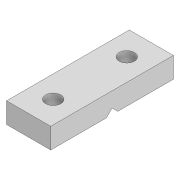
# Autodesk Inventor part: suction_electrode_holder
Saved by Autodesk Inventor 2020 (Build 240168000, 168)
## iProperties
Created: 2020-06-24
Part Number: suction_electrode_holder
Material: Generic
Document SubType Name: Modeling
Designer: Daniel
Density: 1 g/cm^3
Appearance: Default
Author: Daniel
Autodesk Inventor part; units mm, degrees
ref_plane "YZ Plane" through (0, 0, 0) normal (1, 0, 0) x (0, 1, 0)
ref_plane "XZ Plane" through (0, 0, 0) normal (0, 1, 0) x (-1, 0, 0)
ref_plane "XY Plane" through (0, 0, 0) normal (0, 0, 1) x (1, 0, 0)
sketch "Sketch1" plane through (0, 0, 0) normal (0, 1, 0) x (-1, 0, 0)
  line L0 (0, 0) -> (9, 0)
  line L1 (9, 0) -> (9, -25)
  line L2 (9, -25) -> (0, -25)
  line L3 (0, -25) -> (0, 0)
  circle A0 centre (4.5, -5) radius 1.55
  circle A1 centre (4.5, -20) radius 1.55
  line L4 (4.5, 0) -> (4.5, -25) construction
  line L5 (9, -12.5) -> (0, -12.5) construction
  dimension "d0" = 9
  dimension "d1" = 3.1
  dimension "d2" = 3.1
  dimension "d3" = 7.5
  dimension "d4" = 7.5
  dimension "d5" = 25
  constraints: 12 end point, 4 midpoint, 2 centre point, 2 parallel, 1 horizontal, 1 perpendicular, 1 point on line, 1 vertical alignment
  measures "d0" distance of L1.end L2.end
  measures "d1" diameter of A0
  measures "d2" diameter of A1
  measures "d3" distance from line of L5 A0.centre
  measures "d4" distance from line of L5 A1.centre
  measures "d5" distance of L0.end L1.end
extrude "Extrusion1" add sketch "Sketch1" along normal blind 4.2
sketch "Sketch2" plane through (0, 0, 0) normal (1, 0, 0) x (0, 0, -1)
  line L0 (0, 0) -> (25, 0) construction
  line L1 (12.5, 0) -> (12.5, 1.1571) construction
  line L2 (12.5, 1.1571) -> (11.3429, 0)
  line L3 (12.5, 1.1571) -> (13.6571, 0)
  line L4 (9.1461, 0) -> (13.6571, 0)
  circle A0 centre (12.5, 0.45) radius 0.5
  point P0 (11.3429, 0)
  dimension "d8" = 45
  dimension "d10" = 45
  dimension "d14" = 1
  dimension "d15" = 0.45
  constraints: 8 end point, 3 point on line, 1 centre point, 1 collinear, 1 midpoint, 1 tangent, 1 vertical
  measures "d8" angle of L2 L1
  measures "d10" angle of L1 L3
  measures "d14" diameter of A0
  measures "d15" distance from line of L0 A0.centre
extrude "Extrusion2" cut sketch "Sketch2" against normal through all contours L3 A0 L2 | A0 L4 L2 | A0 L4 | L3 L4 A0 picked at (12.3997, 0.4044)
equation "\"d1\" = d2"
equation "\"d4\" = d3"
equation "\"d10\" = d8"
body "Solid1"
